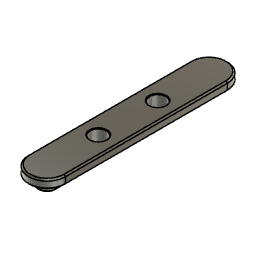
Fixated clamp (Autodesk Fusion 360 design; units mm, degrees)
Autodesk Fusion 360 part; units mm, degrees
note: some values were not read from the file. Set by a fixed rule: which sketch regions a step uses.
sketch "Sketch1" plane through (0, 0, 0) normal (0, 0, 1) x (1, 0, 0)
  circle A0 centre (0, 0) radius 3.15
  circle A1 centre (0, 54.5) radius 3.15
  line L0 (3.15, 0) -> (3.15, 54.5)
  line L1 (-3.15, 54.5) -> (-3.15, 55.0518)
  line L2 (-3.15, 55.0518) -> (-3.15, 0)
  dimension "d2" = 6.3
  dimension "d3" = 54.5
  constraint coincident A0.centre origin
  constraint coincident A0 L0.start
  constraint coincident A1 L0.end
  constraint tangent A1 L0
  constraint coincident A1 L1.start
  constraint parallel L0 L1
  constraint coincident A0 L2.end
  constraint tangent A0 L2
  constraint tangent A0 L0
  constraint tangent A1 L2
  constraint vertical A0.centre A1.centre
  constraint equal A0 A1
  measures "d2" diameter of A1
  measures "d3" distance of A0.centre A1.centre
extrude "Extrude1" add sketch "Sketch1" along normal blind 3
sketch "Sketch2" plane through (0, 0, 3) normal (0, 0, 1) x (-1, 0, 0)
  line L0 (3.15, -54.5) -> (3.15, 0)
  arc A0 (3.15, 0) -> (-3.15, 0) centre (0, 0) ccw
  line L1 (-3.15, 0) -> (-3.15, -54.5)
  arc A1 (-3.15, -54.5) -> (3.15, -54.5) centre (0, -54.5) ccw
  line L2 (6.2, -54.5) -> (6.2, 0)
  arc A2 (6.2, 0) -> (-6.2, 0) centre (0, 0) ccw
  line L3 (-6.2, 0) -> (-6.2, -54.5)
  arc A3 (-6.2, -54.5) -> (6.2, -54.5) centre (0, -54.5) ccw
  arc A4 (-3.15, -54.5) -> (3.15, -54.5) centre (0, -54.5) ccw
  line L4 (-3.15, -54.5) -> (-3.15, 0)
  arc A5 (3.15, 0) -> (-3.15, 0) centre (0, 0) ccw
  line L5 (3.15, 0) -> (3.15, -54.5)
  constraint concentric A0 A2
  constraint concentric A1 A3
  constraint tangent L2 A2
  constraint tangent L3 A3
  constraint tangent A2 L3
  constraint tangent L2 A3
extrude "Extrude2" add sketch "Sketch2" along normal blind 3 contours L0 A0 L1 A1 A4 L4 A5 L5 | L2 A2 L3 A3
chamfer "Chamfer1" distance 0.5 angle 45 12 edges at (6.2, 27.25, 6) (0, 60.7, 6) (-6.2, 27.25, 6) (0, -6.2, 6) (6.2, 27.25, 3) (0, 60.7, 3) (-6.2, 27.25, 3) (0, -6.2, 3) (3.15, 27.25, 0) (0, 57.65, 0) (-3.15, 27.25, 0) (0, -3.15, 0)
sketch "Sketch3" plane through (0, 0, 6) normal (0, 0, 1) x (-1, 0, 0)
  line L0 (-5.7, 0) -> (-5.7, -54.5)
  arc A0 (-5.7, -54.5) -> (5.7, -54.5) centre (0, -54.5) ccw
  line L1 (5.7, -54.5) -> (5.7, 0)
  arc A1 (5.7, 0) -> (-5.7, 0) centre (0, 0) ccw
  point P0 (0, -27.25)
  point P1 (-5.7, -27.25)
  point P2 (0, -37.25)
  point P3 (0, -17.25)
  dimension "d11" = 10
  dimension "d12" = 10
  constraint vertical A0.centre P0
  constraint midpoint L0 P1
  constraint horizontal P0 P1
  constraint vertical P0 P2
  constraint vertical P0 P3
  measures "d11" distance of P0 P3
  measures "d12" distance of P0 P2
hole "Hole1" at (0, 37.25, 6) at (0, 17.25, 6) direction (0, 0, -1) diameter 5.5 end up to surface (6 mm away)
chamfer "Chamfer2" distance 0.2 angle 45 2 edges at (-2.5639, 18.2444, 6) (-2.5639, 38.2444, 6)
chamfer "Chamfer3" distance 0.2 angle 45 8 edges at (0, 20, 0) (0, 14.5, 0) (-2.75, 17.25, 0.1) (2.75, 17.25, 0.1) (0, 34.5, 0) (2.75, 37.25, 0.1) (0, 40, 0) (-2.75, 37.25, 0.1)
